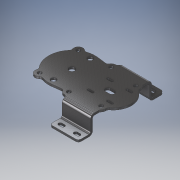
# Autodesk Inventor part: SIDE REDUCTION PLATE II (PLEGADO)
Saved by Autodesk Inventor 2017 (Build 210142000, 142)
## iProperties
Part Number: SIDE REDUCTION PLATE II (PLEGADO)
Material: Genérico
Document SubType Name: Modeling
Designer: Cristian
Density: 1 g/cm^3
Appearance: Valor por defecto
Author: Cristian
Autodesk Inventor part; units mm, degrees
ref_plane "XZ Plane" through (0, 0, 0) normal (0, 1, 0) x (-1, 0, 0)
ref_plane "XY Plane" through (0, 0, 0) normal (0, 0, 1) x (1, 0, 0)
sketch "Boceto1" plane through (0, 0, 0) normal (0, 0, 1) x (1, 0, 0)
  circle A0 centre (0, 0) radius 57.15
  circle A1 centre (101.6, 0) radius 44.45
  circle A2 centre (-31.75, 47.519) radius 11.1125
  circle A3 centre (-31.75, -47.519) radius 11.1125
  circle A4 centre (114.3, 42.5971) radius 11.1125
  circle A5 centre (114.3, -42.5971) radius 11.1125
  line L0 (7.1437, 56.7018) -> (107.1562, 44.1014)
  circle A6 centre (44.45, 52.0016) radius 11.1125
  line L1 (7.1437, -56.7018) -> (107.1562, -44.1014)
  circle A7 centre (44.45, -52.0016) radius 11.1125
  dimension "d0" = 114.3
  dimension "d1" = 88.9
  dimension "d2" = 203.2
  dimension "d3" = 22.225
  dimension "d4" = 22.225
  dimension "d7" = 22.225
  dimension "d8" = 22.225
  dimension "d11" = 22.225
  dimension "d13" = 0
  dimension "d14" = 22.225
  dimension "d35" = 31.75
  dimension "d36" = 31.75
  dimension "d37" = 44.45
  dimension "d38" = 44.45
  dimension "d39" = 12.7
  dimension "d40" = 12.7
  constraints: 8 centre point, 8 point on circle, 4 end point, 4 tangent, 2 point on line, 1 coincident
  measures "d0" diameter of A0
  measures "d1" diameter of A1
  measures "d3" diameter of A2
  measures "d4" diameter of A3
  measures "d7" diameter of A4
  measures "d8" diameter of A5
  measures "d11" diameter of A6
  measures "d13" vertical distance of point (0, 0) A1.centre
  measures "d14" diameter of A7
  measures "d35" horizontal distance of A0.centre A3.centre
  measures "d36" horizontal distance of A0.centre A2.centre
  measures "d37" horizontal distance of point (0, 0) A7.centre
  measures "d38" horizontal distance of point (0, 0) A6.centre
  measures "d39" horizontal distance of A1.centre A5.centre
  measures "d40" horizontal distance of A1.centre A4.centre
extrude "Extrusión1" add sketch "Boceto1" along normal blind 5
ref_plane "Plano de trabajo1" through (50.8, 0, 0) normal (1, 0, 0) x (0, 1, 0)
sketch "Boceto3" plane through (50.8, 0, 0) normal (1, 0, 0) x (0, 1, 0)
  line L0 (-52.7651, 5) -> (-56.7018, 5) projected
  line L1 (0, 0) -> (69.85, 0)
  line L2 (69.85, 0) -> (69.85, -39.45)
  line L3 (58.6315, 5) -> (40.4764, 5) projected
  line L4 (69.85, -39.45) -> (104.775, -39.45)
  line L5 (104.775, -39.45) -> (104.775, -34.45)
  line L6 (104.775, -34.45) -> (74.85, -34.45)
  line L7 (74.85, -34.45) -> (74.85, 5)
  line L8 (74.85, 5) -> (0, 5)
  line L9 (40.4764, 5) -> (-40.4764, 5) projected
  line L10 (0, 0) -> (0, 5)
  point P0 (-54.7334, 5)
  point P1 (-37.2916, 4.445)
  point P2 (52.7651, 5)
  dimension "d123" = 69.85
  dimension "d124" = 44.45
  dimension "d125" = 104.775
  dimension "d126" = 5
  dimension "d127" = 5
  constraints: 16 end point, 4 perpendicular, 2 horizontal, 1 midpoint, 1 vertical, 2 other
  measures "d123" distance of L1.start L1.end
  measures "d124" distance from line of L3 L2.end
  measures "d125" horizontal distance of L1.start L4.end
  measures "d126" distance between parallel lines of L2 L7
  measures "d127" distance between parallel lines of L6 L4
extrude "Extrusión3" add sketch "Boceto3" along normal blind 69.85
mirror "Simetría1" about plane through (0, 0, 0) normal (0, 1, 0) of "Extrusión3"
sketch "Boceto2" plane through (0, 0, 5) normal (0, 0, 1) x (1, 0, 0)
  arc A0 (-21.9537, 52.7651) -> (-40.3458, 40.4764) centre (-31.75, 47.519) ccw projected
  circle A1 centre (-31.75, 47.519) radius 4.7625
  arc A2 (-40.3458, -40.4764) -> (-21.9537, -52.7651) centre (-31.75, -47.519) ccw projected
  circle A3 centre (-31.75, -47.519) radius 4.7625
  arc A4 (33.4247, -53.3907) -> (55.4753, -50.6125) centre (44.45, -52.0016) ccw projected
  circle A5 centre (44.45, -52.0016) radius 4.7625
  arc A6 (55.4753, 50.6125) -> (33.4247, 53.3907) centre (44.45, 52.0016) ccw projected
  circle A7 centre (44.45, 52.0016) radius 4.7625
  arc A8 (124.4689, 38.1158) -> (103.3657, 44.5789) centre (114.3, 42.5971) ccw projected
  circle A9 centre (114.3, 42.5971) radius 4.7625
  arc A10 (103.3657, -44.5789) -> (124.4689, -38.1158) centre (114.3, -42.5971) ccw projected
  circle A11 centre (114.3, -42.5971) radius 4.7625
  point P0 (0, 0)
  dimension "d18" = 9.525
  dimension "d19" = 9.525
  dimension "d20" = 9.525
  dimension "d21" = 9.525
  dimension "d22" = 9.525
  dimension "d23" = 9.525
  constraints: 6 centre point, 6 coincident
  measures "d18" diameter of A1
  measures "d19" diameter of A3
  measures "d20" diameter of A5
  measures "d21" diameter of A7
  measures "d22" diameter of A9
  measures "d23" diameter of A11
extrude "Extrusión2" cut sketch "Boceto2" against normal up to surface (5 mm away)
fillet "Empalme6" radius 6.35 12 edges at (124.4689, 38.1158, 2.5) (120.65, 51.7166, 2.5) (-40.3458, 40.4764, 2.5) (-21.9537, 52.7651, 2.5) (124.4689, -38.1158, 2.5) (120.65, -51.7166, 2.5) (-21.9537, -52.7651, 2.5) (-40.3458, -40.4764, 2.5) (33.4247, -53.3907, 2.5) (50.8, -61.1211, 2.5) (50.8, 61.1211, 2.5) (33.4247, 53.3907, 2.5)
sketch "Boceto5" plane through (0, 0, 5) normal (0, 0, 1) x (1, 0, 0)
  circle A0 centre (0, 0) radius 7.1437
  line L0 (0, 0) -> (0, 45)
  line L1 (0, 0) -> (0, -45)
  circle A1 centre (0, 45) radius 6.35
  circle A2 centre (0, -45) radius 6.35
  dimension "d58" = 14.2875
  dimension "d59" = 45
  dimension "d60" = 45
  dimension "d61" = 12.7
  dimension "d62" = 12.7
  constraints: 4 end point, 3 centre point, 3 coincident, 2 vertical
  measures "d58" diameter of A0
  measures "d59" distance of L0.start L0.end
  measures "d60" distance of L0.start L1.end
  measures "d61" diameter of A1
  measures "d62" diameter of A2
extrude "Extrusión5" cut sketch "Boceto5" against normal up to surface (5 mm away)
sketch "Boceto6" plane through (0, 0, 5) normal (0, 0, 1) x (1, 0, 0)
  circle A0 centre (93.4212, 0) radius 6.35
  circle A1 centre (88.2618, 0) radius 6.35
  circle A2 centre (98.5806, 0) radius 6.35
  line L0 (88.2618, 6.35) -> (98.5806, 6.35)
  line L1 (98.5806, -6.35) -> (88.2618, -6.35)
  line L2 (69.6712, 23.75) -> (117.1712, 23.75)
  line L3 (117.1712, 23.75) -> (117.1712, -23.75)
  line L4 (117.1712, -23.75) -> (69.6712, -23.75)
  line L5 (69.6712, -23.75) -> (69.6712, 23.75)
  circle A3 centre (74.8306, 23.75) radius 2.7781
  circle A4 centre (64.5118, 23.75) radius 2.7781
  line L6 (74.8306, 26.5281) -> (64.5118, 26.5281)
  line L7 (64.5118, 20.9719) -> (74.8306, 20.9719)
  circle A5 centre (74.8306, -23.75) radius 2.7781
  circle A6 centre (64.5118, -23.75) radius 2.7781
  line L8 (64.5118, -20.9719) -> (74.8306, -20.9719)
  line L9 (74.8306, -26.5281) -> (64.5118, -26.5281)
  circle A7 centre (112.0118, -23.75) radius 2.7781
  circle A8 centre (122.3306, -23.75) radius 2.7781
  line L10 (112.0118, -20.9719) -> (122.3306, -20.9719)
  line L11 (112.0118, -26.5281) -> (122.3306, -26.5281)
  circle A9 centre (112.0118, 23.75) radius 2.7781
  circle A10 centre (122.3306, 23.75) radius 2.7781
  line L12 (112.0118, 26.5281) -> (122.3306, 26.5281)
  line L13 (112.0118, 20.9719) -> (122.3306, 20.9719)
  point P0 (0, 0)
  dimension "d65" = 12.7
  dimension "d66" = 0
  dimension "d67" = 93.4212
  dimension "d68" = 12.7
  dimension "d69" = 12.7
  dimension "d70" = 5.1594
  dimension "d71" = 5.1594
  dimension "d72" = 47.5
  dimension "d73" = 47.5
  dimension "d74" = 23.75
  dimension "d75" = 23.75
  dimension "d76" = 5.5563
  dimension "d77" = 5.5563
  dimension "d78" = 5.1594
  dimension "d79" = 5.1594
  dimension "d80" = 0
  dimension "d81" = 5.5563
  dimension "d82" = 5.5563
  dimension "d83" = 5.1594
  dimension "d84" = 5.1594
  dimension "d85" = 0
  dimension "d86" = 0
  dimension "d87" = 5.5563
  dimension "d88" = 5.5563
  dimension "d89" = 5.1594
  dimension "d90" = 5.1594
  dimension "d91" = 0
  dimension "d92" = 5.5563
  dimension "d93" = 5.5563
  dimension "d94" = 5.1594
  dimension "d95" = 5.1594
  dimension "d96" = 0
  constraints: 28 end point, 20 point on circle, 20 tangent, 11 centre point, 4 point on line, 2 horizontal, 2 parallel, 1 perpendicular
  measures "d65" diameter of A0
  measures "d66" vertical distance of point (0, 0) A0.centre
  measures "d67" distance of point (0, 0) A0.centre
  measures "d68" diameter of A1
  measures "d69" diameter of A2
  measures "d70" distance of A0.centre A1.centre
  measures "d71" distance of A0.centre A2.centre
  measures "d72" distance of L2.start L2.end
  measures "d73" distance of L2.end L3.end
  measures "d74" distance from line of A0.centre L3
  measures "d75" distance from line of L2 A0.centre
  measures "d76" diameter of A3
  measures "d77" diameter of A4
  measures "d78" distance of A4.centre L2.start
  measures "d79" distance of L2.start A3.centre
  measures "d80" vertical distance of A3.centre A4.centre
  measures "d81" diameter of A5
  measures "d82" diameter of A6
  measures "d83" distance of L4.end A5.centre
  measures "d84" distance of L4.end A6.centre
  measures "d85" distance from line of L4 A6.centre
  measures "d86" vertical distance of A0.centre A2.centre
  measures "d87" diameter of A7
  measures "d88" diameter of A8
  measures "d89" distance of L3.end A7.centre
  measures "d90" distance of L3.end A8.centre
  measures "d91" vertical distance of A7.centre A8.centre
  measures "d92" diameter of A9
  measures "d93" diameter of A10
  measures "d94" distance of L2.end A9.centre
  measures "d95" distance of A10.centre L2.end
  measures "d96" vertical distance of A9.centre A10.centre
extrude "Extrusión6" cut sketch "Boceto6" against normal up to next contours A0 A2 A1 | A0 A2 | A2 A1 A0 | A0 L0 A2 | A2 L1 A0 | A0 A1 A2 | A0 A1 L0 | A2 A1 A0 | A1 A2 | L1 A1 A0 | A0 A1 | A9 L12 A10 L13 L3 L2 | A9 L2 | L2 A9 | L2 L3 L13 A9 | A3 L2 | L2 A3 | A10 | L10 A8 L11 A7 L4 L3 | L3 L4 A7 L10 | A3 L7 L5 L2 | L2 L5 L7 A4 L6 A3 | A7 L4 | A8 | A4 | A7 L4 | L8 A5 L4 L5 | L5 L4 A5 L9 A6 L8 | A5 L4 | L4 A5 | A6
fillet "Empalme7" radius 4.445 4 edges at (85.725, 74.85, -34.45) (85.725, 69.85, 0) (85.725, -69.85, 0) (85.725, -74.85, -34.45)
fillet "Empalme8" radius 8.89 4 edges at (85.725, 69.85, -39.45) (85.725, -69.85, -39.45) (85.725, -74.85, 5) (85.725, 74.85, 5)
fillet "Empalme9" radius 6.35 4 edges at (120.65, 104.775, -36.95) (50.8, 104.775, -36.95) (120.65, -104.775, -36.95) (50.8, -104.775, -36.95)
sketch "Boceto8" plane through (50.8, 79.295, -34.45) normal (0, 0, 1) x (1, 0, 0)
  circle A0 centre (15.875, 12.78) radius 4.3656
  line L0 (0, 19.13) -> (0, 0) projected
  circle A1 centre (12.5016, 12.78) radius 4.3656
  circle A2 centre (19.2484, 12.78) radius 4.3656
  line L1 (19.2484, 12.78) -> (15.875, 12.78)
  line L2 (15.875, 12.78) -> (12.5016, 12.78)
  line L3 (19.2484, 17.1456) -> (12.5016, 17.1456)
  line L4 (19.2484, 8.4144) -> (12.5016, 8.4144)
  line L5 (6.35, 25.48) -> (63.5, 25.48) projected
  circle A3 centre (57.3484, 12.78) radius 4.3656
  circle A4 centre (53.975, 12.78) radius 4.3656
  circle A5 centre (50.6016, 12.78) radius 4.3656
  line L6 (69.85, 19.13) -> (69.85, 0) projected
  line L7 (57.3484, 12.78) -> (53.975, 12.78)
  line L8 (53.975, 12.78) -> (50.6016, 12.78)
  line L9 (57.3484, 17.1456) -> (50.6016, 17.1456)
  line L10 (57.3484, 8.4144) -> (50.6016, 8.4144)
  point P0 (-50.8, -79.295)
  dimension "d131" = 8.7312
  dimension "d132" = 15.875
  dimension "d133" = 8.7312
  dimension "d134" = 8.7312
  dimension "d135" = 3.3734
  dimension "d136" = 12.7
  dimension "d137" = 8.7312
  dimension "d138" = 8.7312
  dimension "d139" = 8.7312
  dimension "d140" = 12.7
  dimension "d141" = 15.875
  constraints: 16 end point, 8 point on circle, 6 centre point, 4 equal length, 4 horizontal, 4 tangent, 3 collinear
  measures "d131" diameter of A0
  measures "d132" distance from line of L0 L1.end
  measures "d133" diameter of A1
  measures "d134" diameter of A2
  measures "d135" distance of L2.end L1.end
  measures "d136" distance from line of L5 L1.end
  measures "d137" diameter of A3
  measures "d138" diameter of A4
  measures "d139" diameter of A5
  measures "d140" distance from line of L5 L7.end
  measures "d141" distance from line of L6 L7.end
extrude "Extrusión8" cut sketch "Boceto8" against normal up to next
mirror "Simetría3" about plane through (0, 0, 0) normal (0, 1, 0) of "Extrusión8"
equation "\"d16\" = t"
equation "\"d18\" = Q"
equation "\"d19\" = Q"
equation "\"d20\" = Q"
equation "\"d21\" = Q"
equation "\"d22\" = Q"
equation "\"d23\" = Q"
equation "\"d58\" = DF"
equation "\"d59\" = 0.5 * JF"
equation "\"d60\" = 0.5 * JF"
equation "\"d61\" = NF"
equation "\"d62\" = NF"
equation "\"d65\" = DM"
equation "\"d67\" = CM"
equation "\"d68\" = DM"
equation "\"d69\" = DM"
equation "\"d72\" = BM"
equation "\"d73\" = BM"
equation "\"d74\" = 0.5 * BM"
equation "\"d75\" = 0.5 * BM"
equation "\"d76\" = NM"
equation "\"d77\" = NM"
equation "\"d81\" = NM"
equation "\"d82\" = NM"
equation "\"d87\" = NM"
equation "\"d88\" = NM"
equation "\"d92\" = NM"
equation "\"d93\" = NM"
equation "\"t\" = 5"
equation "\"Q\" = 9.525"
equation "\"DF\" = 14.2875"
equation "\"NF\" = 12.7"
equation "\"DH\" = 8.73125"
equation "\"DM\" = 12.7"
equation "\"NM\" = 5.55625"
equation "\"CM\" = 93.4212"
equation "\"AM\" = 56"
equation "\"BM\" = 47.5"
equation "\"JF\" = 90"
